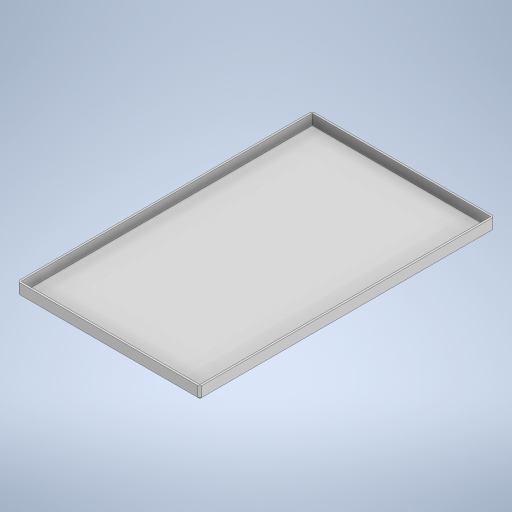
# Autodesk Inventor part: test
Saved by Autodesk Inventor 2024 (Build 280153000, 153)
## iProperties
Created: 2023-10-09
Part Number: test
Material: 常规
Document SubType Name: Modeling
Designer: Administrator
Density: 1 g/cm^3
Appearance: 默认
Author: Administrator
Autodesk Inventor part; units mm, degrees
ref_plane "YZ Plane" through (0, 0, 0) normal (1, 0, 0) x (0, 1, 0)
ref_plane "XZ Plane" through (0, 0, 0) normal (0, 1, 0) x (-1, 0, 0)
ref_plane "XY Plane" through (0, 0, 0) normal (0, 0, 1) x (1, 0, 0)
sketch "草图1" plane through (0, 0, 0) normal (0, 1, 0) x (-1, 0, 0)
  line L0 (0, 0) -> (-195, 0)
  line L1 (-195, 0) -> (-195, -315)
  line L2 (-195, -315) -> (0, -315)
  line L3 (0, -315) -> (0, 0)
  dimension "d0" = 195
  dimension "d1" = 315
  constraints: 8 end point, 2 parallel, 1 horizontal, 1 perpendicular
  measures "d0" distance of L2.end L1.end
  measures "d1" distance of L1.end L0.end
extrude "拉伸1" add sketch "草图1" along normal blind 13
shell "抽壳1" thickness 2 removed faces 1 at (65, 13, -210)
chamfer "倒角1" distance 2 angle 45 8 edges at (97.5, 0, 0) (0, 0, -157.5) (195, 0, -157.5) (97.5, 0, -315) (195, 6.5, -315) (195, 6.5, 0) (0, 6.5, 0) (0, 6.5, -315)
